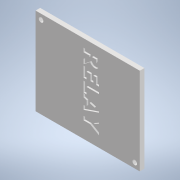
# Autodesk Inventor part: RelayTray
Saved by Autodesk Inventor 2022.2 (Build 262287000, 287)
## iProperties
Created: 2022-01-15
Part Number: RelayTray
Material: Generic
Document SubType Name: Modeling
Designer: siwat
Density: 1 g/cm^3
Appearance: Default
Author: siwat
Autodesk Inventor part; units mm, degrees
ref_plane "YZ Plane" through (0, 0, 0) normal (1, 0, 0) x (0, 1, 0)
ref_plane "XZ Plane" through (0, 0, 0) normal (0, 1, 0) x (-1, 0, 0)
ref_plane "XY Plane" through (0, 0, 0) normal (0, 0, 1) x (1, 0, 0)
ref_plane "Work Plane1" through (-62.4151, 1.9295, 0) normal (0, 0, 1) x (1, 0, 0)
sketch "Sketch1" plane through (-62.4151, 1.9295, 0) normal (0, 0, 1) x (1, 0, 0)
  line L0 (-5.0959, -1.798) -> (62.2123, -1.798)
  line L1 (62.2123, -1.798) -> (62.2123, 54.509)
  line L2 (62.2123, 54.509) -> (-5.0959, 54.509)
  line L3 (-5.0959, 54.509) -> (-5.0959, -1.798)
  circle A0 centre (58.9363, 1.5668) radius 1.5
  circle A1 centre (-1.5532, 51.0932) radius 1.5
  point P0 (62.4151, -1.9295)
  dimension "d0" = 3
  dimension "d1" = 3
  constraints: 8 end point, 2 centre point, 2 parallel, 1 horizontal, 1 perpendicular
  measures "d0" diameter of A0
  measures "d1" diameter of A1
extrude "Extrusion1" add sketch "Sketch1" along normal blind 3
sketch "Sketch2" plane through (-62.4151, 1.9295, 3) normal (0, 0, 1) x (1, 0, 0)
  line L0 (35.8804, 50.2555) -> (35.8804, 5.3448) construction
  line L1 (35.8804, 5.3448) -> (24.8368, 5.3448) construction
  line L2 (24.8368, 5.3448) -> (24.8368, 50.2555) construction
  line L3 (24.8368, 50.2555) -> (35.8804, 50.2555) construction
  line L4 (25.8804, 39.9799) -> (25.8804, 43.035)
  line L5 (25.8804, 43.035) -> (29.5514, 45.8146)
  line L6 (29.5514, 45.8146) -> (29.5514, 46.7222)
  line L7 (29.5514, 46.7222) -> (25.8804, 46.7222)
  line L8 (25.8804, 46.7222) -> (25.8804, 49.2182)
  line L9 (25.8804, 49.2182) -> (35.8804, 49.2182)
  line L10 (35.8804, 49.2182) -> (35.8804, 45.1987)
  spline S0 degree 2 poles (35.8804, 45.1987) (35.8804, 44.3641) (35.6697, 43.1323) (35.3456, 42.6055) knots 0 0 0 1 2 2 2
  spline S1 degree 2 poles (35.3456, 42.6055) (35.0052, 42.0707) (33.9436, 41.4386) (33.1333, 41.4386) knots 0 0 0 1 2 2 2
  spline S2 degree 2 poles (33.1333, 41.4386) (31.9906, 41.4386) (30.5563, 42.4759) (30.1349, 43.343) knots 0 0 0 1 2 2 2
  line L11 (30.1349, 43.343) -> (25.8804, 39.9799)
  spline S3 degree 2 poles (32.8172, 44.0156) (33.1981, 44.0156) (33.741, 44.3073) (33.8869, 44.6396) knots 0 0 0 1 2 2 2
  spline S4 degree 2 poles (33.8869, 44.6396) (33.9842, 44.8746) (34.0409, 45.45) (34.0409, 45.8795) knots 0 0 0 1 2 2 2
  line L12 (34.0409, 45.8795) -> (34.0409, 46.7222)
  line L13 (34.0409, 46.7222) -> (31.3504, 46.7222)
  line L14 (31.3504, 46.7222) -> (31.3504, 46.001)
  spline S5 degree 2 poles (31.3504, 46.001) (31.3504, 45.4824) (31.4801, 44.7449) (31.6827, 44.4937) knots 0 0 0 1 2 2 2
  spline S6 degree 2 poles (31.6827, 44.4937) (31.8772, 44.2506) (32.3958, 44.0156) (32.8172, 44.0156) knots 0 0 0 1 2 2 2
  line L15 (25.8804, 39.2344) -> (35.8804, 39.2344)
  line L16 (35.8804, 39.2344) -> (35.8804, 32.4759)
  line L17 (35.8804, 32.4759) -> (33.9761, 32.4759)
  line L18 (33.9761, 32.4759) -> (33.9761, 36.7384)
  line L19 (33.9761, 36.7384) -> (32.2175, 36.7384)
  line L20 (32.2175, 36.7384) -> (32.2175, 32.8081)
  line L21 (32.2175, 32.8081) -> (30.3132, 32.8081)
  line L22 (30.3132, 32.8081) -> (30.3132, 36.7384)
  line L23 (30.3132, 36.7384) -> (27.7848, 36.7384)
  line L24 (27.7848, 36.7384) -> (27.7848, 32.4759)
  line L25 (27.7848, 32.4759) -> (25.8804, 32.4759)
  line L26 (25.8804, 32.4759) -> (25.8804, 39.2344)
  line L27 (25.8804, 24.1047) -> (25.8804, 30.7741)
  line L28 (25.8804, 30.7741) -> (35.8804, 30.7741)
  line L29 (35.8804, 30.7741) -> (35.8804, 28.262)
  line L30 (35.8804, 28.262) -> (27.7848, 28.262)
  line L31 (27.7848, 28.262) -> (27.7848, 24.1047)
  line L32 (27.7848, 24.1047) -> (25.8804, 24.1047)
  line L33 (25.8804, 23.9832) -> (35.8804, 20.6039)
  line L34 (35.8804, 20.6039) -> (35.8804, 17.8649)
  line L35 (35.8804, 17.8649) -> (25.8804, 14.4856)
  line L36 (25.8804, 14.4856) -> (25.8804, 17.0707)
  line L37 (25.8804, 17.0707) -> (27.9226, 17.6947)
  line L38 (27.9226, 17.6947) -> (27.9226, 20.8389)
  line L39 (27.9226, 20.8389) -> (25.8804, 21.471)
  line L40 (25.8804, 21.471) -> (25.8804, 23.9832)
  line L41 (29.7378, 18.2457) -> (33.0441, 19.2668)
  line L42 (33.0441, 19.2668) -> (29.7378, 20.296)
  line L43 (29.7378, 20.296) -> (29.7378, 18.2457)
  line L44 (35.8804, 5.1744) -> (30.0539, 8.6266)
  line L45 (30.0539, 8.6266) -> (25.8804, 8.6266)
  line L46 (25.8804, 8.6266) -> (25.8804, 11.1388)
  line L47 (25.8804, 11.1388) -> (29.9323, 11.1388)
  line L48 (29.9323, 11.1388) -> (35.8804, 14.6477)
  line L49 (35.8804, 14.6477) -> (35.8804, 11.7871)
  line L50 (35.8804, 11.7871) -> (32.3148, 9.8341)
  line L51 (32.3148, 9.8341) -> (35.8804, 7.9459)
  line L52 (35.8804, 7.9459) -> (35.8804, 5.1744)
  point P0 (62.4151, -1.9295)
  constraints: 2 other
extrude "Extrusion2" cut sketch "Sketch2" against normal blind 1
body "Solid1"
